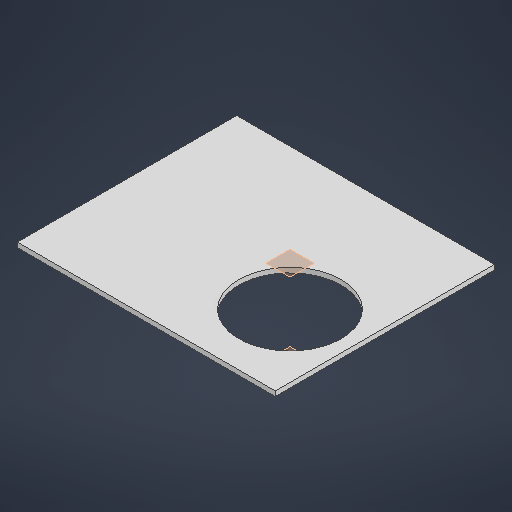
# Autodesk Inventor part: tapa_lanzador_pelota
Saved by Autodesk Inventor 2026.2 (Build 302298010, 298A)
## iProperties
Created: 2026-03-17
Part Number: tapa_lanzador_pelota
Material: Generic
Document SubType Name: Modeling
Designer: trini
Density: 1 g/cm^3
Appearance: Default
Author: trini
Autodesk Inventor part; units mm, degrees
ref_plane "YZ Plane" through (0, 0, 0) normal (1, 0, 0) x (0, 1, 0)
ref_plane "XY Plane" through (0, 0, 0) normal (0, 0, 1) x (1, 0, 0)
ref_plane "Work Plane1" through (0, 35, 0) normal (0, 1, 0) x (-1, 0, 0)
ref_plane "Work Plane2" through (0, -35, 0) normal (0, 1, 0) x (-1, 0, 0)
sketch "Sketch3" plane through (0, 0, 0) normal (0, 1, 0) x (-1, 0, 0)
  line L0 (161.3, -117.07) -> (-52.7, -117.07)
  line L1 (-52.7, -117.07) -> (-52.7, 64.93)
  line L2 (-52.7, 64.93) -> (161.3, 64.93)
  line L3 (161.3, 64.93) -> (161.3, -117.07)
  circle A0 centre (0, 0) radius 37.5
  dimension "d8" = 182
  dimension "d9" = 214
  dimension "d10" = 52.7
  dimension "d11" = 64.93
  dimension "d14" = 75
  constraints: 8 end point, 2 parallel, 1 centre point, 1 coincident, 1 horizontal, 1 perpendicular
  measures "d8" distance of L0.end L1.end
  measures "d9" distance of L1.end L2.end
  measures "d10" distance from line of L1 point (0, 0)
  measures "d11" distance from line of L2 point (0, 0)
  measures "d14" diameter of A0
extrude "Extrusion1" add sketch "Sketch3" along normal mid plane 4
sketch "Sketch4" plane through (0, 35, 0) normal (0, 1, 0) x (-1, 0, 0)
  circle A0 centre (0, 0) radius 37.5
  circle A1 centre (0, 0) radius 42.5
  dimension "d15" = 75
  dimension "d16" = 85
  constraints: 2 centre point, 2 coincident
  measures "d15" diameter of A0
  measures "d16" diameter of A1
extrude "Extrusion2" add sketch "Sketch4" against normal up to surface (70 mm away)
sketch "Sketch5" plane through (0, -35, 0) normal (0, 1, 0) x (-1, 0, 0)
  circle A0 centre (0, 0) radius 37.5
  circle A1 centre (0, 0) radius 20
  dimension "d19" = 75
  dimension "d20" = 40
  constraints: 2 centre point, 2 coincident
  measures "d19" diameter of A0
  measures "d20" diameter of A1
extrude "Extrusion3" add sketch "Sketch5" along normal blind 3
sketch "Sketch6" plane through (0, 0, 0) normal (0, 0, 1) x (1, 0, 0)
  line L0 (-37.5, -32) -> (37.5, -32) projected
  line L1 (-42.5, -35) -> (42.5, -35) projected
  arc A0 (-24.5305, -32) -> (-20, -35) centre (-2.9998, -4.406) ccw
  line L2 (-24.5305, -32) -> (-20, -32)
  line L3 (-20, -35) -> (-20, -32)
  line L4 (-20, -32) -> (-20, -35) projected
  line L5 (-24.5305, -32) -> (-20, -32)
  line L6 (0, -42.1057) -> (0, 7.0176) projected
  point P0 (0, 0)
  dimension "d23" = 35
  dimension "d24" = 4.5305
  constraints: 6 end point, 3 collinear, 3 point on line, 2 point on circle, 1 centre point
  measures "d23" radius of A0
  measures "d24" distance of L2.end L2.start
revolve "Revolution1" cut sketch "Sketch6" angle 360 about axis through (0, -10, 0) along (0, 1, 0) contours L0 L3 A0
sketch "Sketch7" plane through (0, 2, 0) normal (0, 1, 0) x (1, 0, 0)
  circle A0 centre (0, 0) radius 42.5
  circle A1 centre (0, 0) radius 42.5 projected
  dimension "d26" = 85
  constraints: 1 centre point, 1 coincident, 1 concentric
  measures "d26" diameter of A0
extrude "Extrusion4" cut sketch "Sketch7" along normal mid plane 80
body "Solid1"
